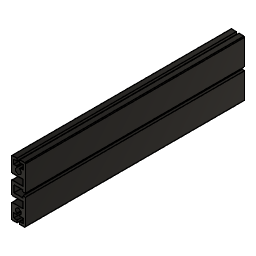
Galaxy_side_panel (Autodesk Fusion 360 design; units mm, degrees)
Autodesk Fusion 360 part; units mm, degrees
sketch "Sketch1" plane through (0, 0, 0) normal (0, 1, 0) x (1, 0, 0)
  line L0 (5, -20) -> (-5, 20) construction
  line L1 (-5, -20) -> (5, 20) construction
  line L2 (-0.965, -18.26) -> (-0.965, -20)
  line L3 (0.965, -20) -> (0.965, -18.26)
  line L4 (0.965, -18.26) -> (0, -20) construction
  line L5 (-0.965, -18.26) -> (0, -20) construction
  line L6 (-5, -18.26) -> (-3.44, -18.26) construction
  line L7 (-0.965, -20) -> (-0.965, -18.26)
  line L8 (0.965, -18.26) -> (0.965, -20)
  line L9 (4.5, -20) -> (0.965, -20)
  line L10 (-0.965, -20) -> (-4.5, -20)
  line L11 (-7.5, 0) -> (8.5, 0)
  line L12 (0, -25) -> (0, 24) construction
  line L13 (5, -18.26) -> (3.44, -18.26) construction
  line L14 (3.44, -18.26) -> (3.44, -15.05)
  line L15 (-3.44, -15.05) -> (-3.44, -18.26)
  line L16 (-3.44, -18.26) -> (-0.965, -18.26)
  line L17 (0.965, -18.26) -> (3.44, -18.26)
  line L18 (-0.965, -18.26) -> (-0.965, -14.5258) construction
  line L19 (0.965, -18.26) -> (0.965, -14.2518) construction
  arc A0 (1.172, -14.1206) -> (-1.172, -14.1206) centre (0, -12.5) ccw
  line L20 (3.44, -15.05) -> (1.465, -15.05)
  line L21 (-1.465, -15.05) -> (-3.44, -15.05)
  line L22 (-0.965, -14.2518) -> (-0.965, -14.55)
  line L23 (0.965, -14.5258) -> (0.965, -14.55)
  arc A1 (-1.465, -15.05) -> (-0.965, -14.55) centre (-1.465, -14.55) ccw
  arc A2 (-0.965, -14.5258) -> (-1.172, -14.1206) centre (-1.465, -14.5258) ccw
  arc A3 (0.965, -14.55) -> (1.465, -15.05) centre (1.465, -14.55) ccw
  arc A4 (1.172, -14.1206) -> (0.965, -14.5258) centre (1.465, -14.5258) ccw
  line L24 (-0.965, 18.26) -> (-0.965, 14.5258) construction
  line L25 (-1.465, 15.05) -> (-3.44, 15.05)
  line L26 (3.44, 18.26) -> (3.44, 15.05)
  arc A5 (1.465, 15.05) -> (0.965, 14.55) centre (1.465, 14.55) ccw
  line L27 (0.965, 18.26) -> (0, 20) construction
  arc A6 (-1.172, 14.1206) -> (1.172, 14.1206) centre (0, 12.5) ccw
  line L28 (-5, 18.26) -> (-3.44, 18.26) construction
  line L29 (3.44, 15.05) -> (1.465, 15.05)
  line L30 (-0.965, 20) -> (-0.965, 18.26)
  arc A7 (0.965, 14.5258) -> (1.172, 14.1206) centre (1.465, 14.5258) ccw
  line L31 (0.965, 14.5258) -> (0.965, 14.55)
  line L32 (-5, 20) -> (5, -20) construction
  line L33 (0.965, 18.26) -> (3.44, 18.26)
  arc A8 (-0.965, 14.55) -> (-1.465, 15.05) centre (-1.465, 14.55) ccw
  line L34 (-0.965, 14.2518) -> (-0.965, 14.55)
  line L35 (5, 18.26) -> (3.44, 18.26) construction
  line L36 (5, 20) -> (-5, -20) construction
  line L37 (0.965, 18.26) -> (0.965, 20)
  line L38 (-3.44, 15.05) -> (-3.44, 18.26)
  line L39 (0.965, 20) -> (0.965, 18.26)
  line L40 (-3.44, 18.26) -> (-0.965, 18.26)
  line L41 (-0.965, 18.26) -> (-0.965, 20)
  line L42 (0.965, 18.26) -> (0.965, 14.2518) construction
  arc A9 (-1.172, 14.1206) -> (-0.965, 14.5258) centre (-1.465, 14.5258) ccw
  line L43 (-0.965, 18.26) -> (0, 20) construction
  line L44 (0, 25) -> (0, -24) construction
  line L45 (-4.5, 20) -> (-0.965, 20)
  line L46 (0.965, 20) -> (4.5, 20)
  line L47 (-5, -20) -> (-5, -9.6) construction
  line L48 (-4.5, -9.1) -> (3.33, -9.1)
  line L49 (3.33, -9.1) -> (3.33, -4.77)
  line L50 (3.33, -4.77) -> (-4.5, -4.77)
  line L51 (-4.5, 9.1) -> (3.33, 9.1)
  line L52 (3.33, 9.1) -> (3.33, 4.77)
  line L53 (3.33, 4.77) -> (-4.5, 4.77)
  line L54 (-5, 9.6) -> (-5, 19.5)
  line L55 (-5, -19.5) -> (-5, -9.1)
  line L56 (-5, -4.27) -> (-5, 4.27)
  line L57 (3.16, -2.5) -> (-3.16, -2.5)
  line L58 (-3.16, -2.5) -> (-3.16, 2.5)
  line L59 (-3.16, 2.5) -> (3.16, 2.5)
  line L60 (3.16, -2.5) -> (-3.16, 2.5) construction
  line L61 (-3.16, -2.5) -> (3.16, 2.5) construction
  line L62 (3.16, 1.225) -> (5, 1.225)
  line L63 (5.66, -1.225) -> (0.66, 1.225) construction
  line L64 (0.66, -1.225) -> (5.66, 1.225) construction
  line L65 (5, 19.5) -> (5, 1.225)
  line L66 (5, -1.225) -> (5, -19.5)
  line L67 (3.16, 2.5) -> (3.16, 1.225)
  line L68 (3.16, -1.225) -> (3.16, -2.5)
  line L69 (5, -1.225) -> (3.16, -1.225)
  arc A10 (4.5, -20) -> (5, -19.5) centre (4.5, -19.5) ccw
  arc A11 (-5, -19.5) -> (-4.5, -20) centre (-4.5, -19.5) ccw
  arc A12 (-4.5, -9.1) -> (-5, -9.6) centre (-4.5, -9.6) ccw
  arc A13 (-5, -4.27) -> (-4.5, -4.77) centre (-4.5, -4.27) ccw
  arc A14 (-4.5, 4.77) -> (-5, 4.27) centre (-4.5, 4.27) ccw
  arc A15 (-5, 9.6) -> (-4.5, 9.1) centre (-4.5, 9.6) ccw
  arc A16 (-4.5, 20) -> (-5, 19.5) centre (-4.5, 19.5) ccw
  arc A17 (5, 19.5) -> (4.5, 20) centre (4.5, 19.5) ccw
  point P0 (-5, -4.77)
  dimension "d1" = 10
  dimension "d2" = 40
  dimension "d5" = 1.56
  dimension "d6" = 1.56
  dimension "d7" = 3.21
  dimension "d9" = 4
  dimension "d10" = 0.5
  dimension "d11" = 0.5
  dimension "d12" = 10.9
  dimension "d13" = 8.33
  dimension "d14" = 4.33
  dimension "d15" = 6.32
  dimension "d16" = 5
  dimension "d17" = 2.45
  dimension "d18" = 0.5
  constraint horizontal L9
  constraint perpendicular L9 L55
  constraint parallel L9 L45
  constraint parallel L55 L65
  constraint coincident L0 origin
  constraint coincident L1 origin
  constraint parallel L2 L3
  constraint coincident L6.start L55
  constraint perpendicular L6 L55
  constraint coincident L2.end L9
  constraint collinear L9 L10
  constraint perpendicular L11 L55
  constraint parallel L12 L55
  constraint coincident L13.start L65
  constraint perpendicular L13 L65
  constraint horizontal L16
  constraint vertical L14
  constraint horizontal L20
  constraint vertical L15
  constraint collinear L16 L17
  constraint perpendicular L16 L18
  constraint perpendicular L17 L19
  constraint collinear L20 L21
  constraint perpendicular L21 L22
  constraint tangent L21 A1
  constraint tangent L22 A1
  constraint coincident L22.start L18
  constraint coincident L22.start A0
  constraint tangent A0 A2
  constraint tangent L18 A2
  constraint equal A1 A2
  constraint tangent L20 A3
  constraint tangent L23 A3
  constraint coincident L19.end L23
  constraint coincident L19.end A0
  constraint tangent L23 A4
  constraint tangent A0 A4
  constraint equal A3 A4
  constraint symmetric L0.start L11 L1.end
  constraint symmetric L1.start L11 L0.end
  constraint symmetric L0.end L11 L1.start
  constraint symmetric L1.end L11 L0.start
  constraint symmetric L3.end L11 L27.start
  constraint symmetric L2.start L11 L24.start
  constraint symmetric L6.start L11 L28.start
  constraint symmetric L6.end L11 L28.end
  constraint symmetric L2.end L11 L30.start
  constraint symmetric L3.start L11 L37.end
  constraint symmetric L11 L12.start L44.start
  constraint symmetric L11 L12.end L44.end
  constraint symmetric L11 L13.start L35.start
  constraint symmetric L11 L13.end L26.start
  constraint symmetric L11 L14.end L26.end
  constraint symmetric L11 L15.start L25.end
  constraint symmetric L11 L22.start L34.start
  constraint symmetric L11 L19.end L42.end
  constraint symmetric L11 A0 A6
  constraint symmetric L11 L4.end L27.end
  constraint symmetric L11 L21.start L25.start
  constraint symmetric L11 L22.end A8.start
  constraint symmetric L11 A1 A8
  constraint symmetric L11 L18.end L24.end
  constraint symmetric L11 A0.end A6.start
  constraint symmetric L11 A2 A9
  constraint symmetric L11 L20.end A5.start
  constraint symmetric L11 L23.end A5.end
  constraint symmetric L11 A3 A5
  constraint symmetric L11 L23.start A7.start
  constraint symmetric L11 A0.start A6.end
  constraint symmetric L11 A4 A7
  constraint collinear L45 L46
  constraint perpendicular L10 L47
  constraint horizontal L48
  constraint vertical L49
  constraint horizontal L50
  constraint symmetric L11 L48.end L51.end
  constraint symmetric L11 L49.end L52.end
  constraint collinear L54 L55
  constraint collinear L55 L56
  constraint horizontal L57
  constraint perpendicular L57 L58
  constraint parallel L57 L59
  constraint parallel L58 L67
  constraint coincident L60 origin
  constraint coincident L61 origin
  constraint horizontal L69
  constraint parallel L62 L69
  constraint coincident L66.start L65
  constraint collinear L65 L66
  constraint collinear L67 L68
  constraint coincident L0.start L9
  constraint coincident L0.start L66
  constraint tangent L9 A10
  constraint tangent L66 A10
  constraint coincident L1.start L55
  constraint coincident L1.start L10
  constraint tangent L55 A11
  constraint tangent L10 A11
  constraint equal A10 A11
  constraint coincident L55.end L48
  constraint tangent L47 A12
  constraint tangent L48 A12
  constraint equal A10 A12
  constraint coincident P0 L56
  constraint coincident P0 L50
  constraint tangent L56 A13
  constraint tangent L50 A13
  constraint equal A10 A13
  constraint tangent L56 A14
  constraint tangent L53 A14
  constraint equal A10 A14
  constraint tangent L54 A15
  constraint tangent L51 A15
  constraint equal A10 A15
  constraint coincident L0.end L45
  constraint coincident L0.end L54
  constraint tangent L45 A16
  constraint tangent L54 A16
  constraint equal A10 A16
  constraint coincident L1.end L46
  constraint coincident L1.end L65
  constraint tangent L46 A17
  constraint tangent L65 A17
  constraint equal A10 A17
  measures "d1" distance of L0.end L1.end
  measures "d2" distance of L1.start L0.end
  measures "d5" distance of L6.start L6.end
  measures "d6" distance of L13.start L13.end
  measures "d7" distance of L6.end L15.start
  measures "d9" diameter of A0
  measures "d10" radius of A1
  measures "d11" radius of A3
  measures "d12" distance of L1.start L55.end
  measures "d13" distance of L55.end L48.end
  measures "d14" distance of L55.end P0
  measures "d15" distance of L58.end L59.end
  measures "d16" distance of L63.end L64.end
  measures "d17" distance of L63.start L64.end
  measures "d18" radius of A10
extrude "Extrude1" add sketch "Sketch1" along normal blind 157
